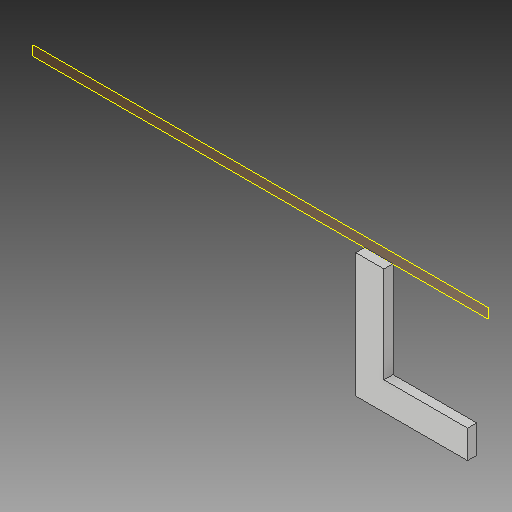
# Autodesk Inventor part: Jig_nodeAirInlet
Saved by Autodesk Inventor 2017 (Build 210142000, 142)
## iProperties
Created: 2017-10-09
Part Number: Jig_nodeAirInlet
Material: Generic
Document SubType Name: Modeling
Designer: Kathryn Rosie
Density: 1 g/cm^3
Appearance: Default
Author: Kathryn Rosie
Autodesk Inventor part; units mm, degrees
ref_plane "YZ Plane" through (0, 0, 0) normal (1, 0, 0) x (0, 1, 0)
ref_plane "XZ Plane" through (0, 0, 0) normal (0, 1, 0) x (-1, 0, 0)
ref_plane "XY Plane" through (0, 0, 0) normal (0, 0, 1) x (1, 0, 0)
ref_plane "Work Plane1" through (-1022, 1522, 0) normal (0, 0, 1) x (1, 0, 0)
sketch "Sketch1" plane through (-1022, 1522, 0) normal (0, 0, 1) x (1, 0, 0)
  line L0 (1022, 22) -> (1022, -1522) projected
  line L1 (1022, 22) -> (1000, 22) projected
  line L2 (1000, -1522) -> (1000, 22) projected
  line L3 (1022, -1522) -> (1000, -1522) projected
  circle A0 centre (880.1401, -150.1401) radius 55 projected
  line L4 (0, 0) -> (1000, 0) projected
  line L5 (1000, 0) -> (1000, 22) projected
  line L6 (0, 22) -> (1000, 22) projected
  line L7 (0, 0) -> (0, 22) projected
  line L8 (752, 0) -> (752, -300)
  line L9 (752, -300) -> (1022, -300)
  line L10 (1022, -300) -> (1022, -232)
  line L11 (1022, -232) -> (820, -232)
  line L12 (820, -232) -> (820, 0)
  line L13 (1022, 22) -> (1000, 22)
  line L14 (820, 0) -> (752, 0)
  line L15 (0, 0) -> (2000, 0) construction
  line L16 (0, 0) -> (2000, 0) construction
  point P0 (1022, -1522)
  dimension "d0" = 270
  dimension "d1" = 300
  dimension "d3" = 232
  dimension "d4" = 202
  dimension "d6" = 2000
  dimension "d8" = 1022
  constraints: 19 end point, 5 horizontal, 4 parallel, 2 perpendicular, 1 collinear, 1 point on line, 1 vertical
  measures "d0" distance of L9.end L8.end
  measures "d1" distance of L8.end L8.start
  measures "d3" distance between parallel lines of L14 L11
  measures "d4" distance between parallel lines of L10 L12
  measures "d6" distance of L4.start L15.end
  measures "d8" distance from line of L4.start L10
extrude "Extrusion1" add sketch "Sketch1" along normal blind 22 contours L0 L9 L2 L11 | L2 L9 L8 L4 L12 L11
body "Solid1"
